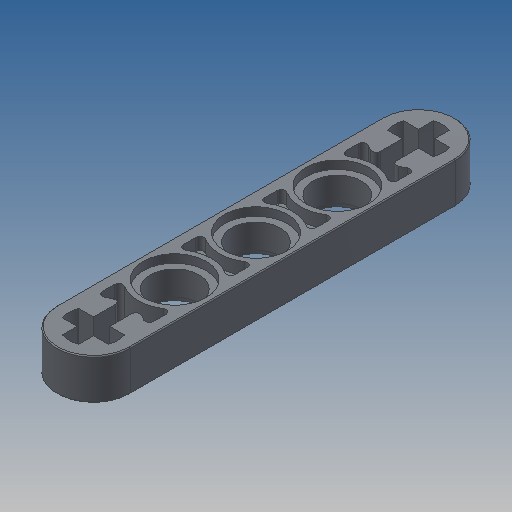
# Autodesk Inventor part: 11478-LtBluishGray
Saved by Autodesk Inventor 2022.2 (Build 262287010, 287A)
## iProperties
Created: 2012-03-21
Part Number: 11478-LtBluishGray
Document SubType Name: Modeling
Designer: D. Kohfeld
Density: 1.06 g/cm^3
Material: ABS Plastic
Mass: 0.640676 g
Surface Area: 12.0343 cm^2
Volume: 0.604411 cm^3
Appearance: LtBluishGray
Author: D. Kohfeld
Autodesk Inventor part; units mm, degrees
ref_plane "YZ Plane" through (0, 0, 0) normal (1, 0, 0) x (0, 1, 0)
ref_plane "XZ Plane" through (0, 0, 0) normal (0, 1, 0) x (-1, 0, 0)
ref_plane "XY Plane" through (0, 0, 0) normal (0, 0, 1) x (1, 0, 0)
sketch "Sketch1" plane through (0, 0, 0) normal (0, 0, 1) x (1, 0, 0)
  line L0 (3.6, -16) -> (3.6, 16)
  line L1 (-3.6, 16) -> (-3.6, -16)
  arc A0 (3.6, 16) -> (-3.6, 16) centre (0, 16) ccw
  circle A1 centre (0, 16) radius 2.4 construction
  circle A2 centre (0, 16) radius 3.2 construction
  circle A3 centre (0, 8) radius 3.2
  circle A4 centre (0, 8) radius 2.4
  line L2 (0, 8) -> (0, 16) construction
  line L3 (-2.5456, 13.4544) -> (-2.5456, 10.5456)
  line L4 (2.5456, 13.4544) -> (2.5456, 10.5456)
  arc A5 (-2.5456, 13.4544) -> (2.5456, 13.4544) centre (0, 16) ccw
  arc A6 (2.5456, 10.5456) -> (-2.5456, 10.5456) centre (0, 8) ccw
  arc A7 (-3.6, -16) -> (3.6, -16) centre (0, -16) ccw
  circle A8 centre (0, -16) radius 3.2 construction
  circle A9 centre (0, -16) radius 2.4 construction
  line L5 (-2.5456, -10.5456) -> (-2.5456, -13.4544)
  line L6 (2.5456, -10.5456) -> (2.5456, -13.4544)
  arc A10 (2.5456, -13.4544) -> (-2.5456, -13.4544) centre (0, -16) ccw
  line L7 (0.8, 12.49) -> (0.8, 15.2)
  line L8 (0.8, 15.2) -> (2.2627, 15.2)
  line L9 (2.2627, 16.8) -> (0.8, 16.8)
  line L10 (0.8, 16.8) -> (0.8, 18.2627)
  line L11 (-0.8, 18.2627) -> (-0.8, 16.8)
  line L12 (-0.8, 16.8) -> (-2.2627, 16.8)
  line L13 (-2.2627, 15.2) -> (-0.8, 15.2)
  line L14 (-0.8, 15.2) -> (-0.8, 12.49)
  arc A11 (-2.2627, 16.8) -> (-2.2627, 15.2) centre (0, 16) ccw
  arc A12 (0.8, 18.2627) -> (-0.8, 18.2627) centre (0, 16) ccw
  arc A13 (2.2627, 15.2) -> (2.2627, 16.8) centre (0, 16) ccw
  line L15 (-0.8, -18.2627) -> (-0.8, -16.8)
  line L16 (-0.8, -16.8) -> (-2.2627, -16.8)
  line L17 (-2.2627, -15.2) -> (-0.8, -15.2)
  line L18 (-0.8, -15.2) -> (-0.8, -12.49)
  line L19 (0.8, -12.49) -> (0.8, -15.2)
  line L20 (0.8, -15.2) -> (2.2627, -15.2)
  line L21 (2.2627, -16.8) -> (0.8, -16.8)
  line L22 (0.8, -16.8) -> (0.8, -18.2627)
  arc A14 (-2.2627, -15.2) -> (-2.2627, -16.8) centre (0, -16) ccw
  arc A15 (-0.8, -18.2627) -> (0.8, -18.2627) centre (0, -16) ccw
  arc A16 (2.2627, -16.8) -> (2.2627, -15.2) centre (0, -16) ccw
  circle A17 centre (0, 0) radius 3.2
  circle A18 centre (0, 0) radius 2.4
  circle A19 centre (0, -8) radius 3.2
  circle A20 centre (0, -8) radius 2.4
  line L23 (0, 8) -> (0, 0) construction
  line L24 (0, 0) -> (0, -8) construction
  line L25 (0, -8) -> (0, -16) construction
  line L26 (-2.5456, 13.4544) -> (0, 16) construction
  arc A21 (-2.5456, -10.5456) -> (2.5456, -10.5456) centre (0, -8) ccw
  line L27 (-2.5456, 5.4544) -> (-2.5456, 2.5456)
  line L28 (-2.5456, -2.5456) -> (-2.5456, -5.4544)
  line L29 (2.5456, -2.5456) -> (2.5456, -5.4544)
  line L30 (2.5456, 5.4544) -> (2.5456, 2.5456)
  arc A22 (-2.5456, 5.4544) -> (2.5456, 5.4544) centre (0, 8) ccw
  arc A23 (2.5456, 2.5456) -> (-2.5456, 2.5456) centre (0, 0) ccw
  arc A24 (-2.5456, -2.5456) -> (2.5456, -2.5456) centre (0, 0) ccw
  arc A25 (2.5456, -5.4544) -> (-2.5456, -5.4544) centre (0, -8) ccw
  dimension "d8" = 4.8
  dimension "d9" = 6.4
  dimension "d32" = 7.2
  dimension "d34" = 8
  dimension "d52" = 1.6
  dimension "d54" = 45
  constraints: 62 end point, 48 point on circle, 26 centre point, 23 equal radius, 18 equal length, 17 coincident, 14 parallel, 7 perpendicular, 7 vertical alignment, 5 collinear, 4 tangent, 3 vertical
  measures "d8" diameter of A1
  measures "d9" diameter of A2
  measures "d32" diameter of A0
  measures "d34" distance of L2.start L2.end
  measures "d52" distance between parallel lines of L10 L11
  measures "d54" angle of L1 L26
extrude "Extrusion1" add sketch "Sketch1" along normal mid plane 4 contours A7 L1 A0 L0 | A3 | A17 | A19
extrude "Extrusion9" add sketch "Sketch1" along normal mid plane 1.6 contours A22 L30 A23 L27 | A24 L29 A25 L28
sketch "Sketch6" plane through (0, 0, 2) normal (0, 0, 1) x (1, 0, 0)
  circle A0 centre (0, 8) radius 3.1
  circle A1 centre (0, 8) radius 2.4 projected
  arc A2 (2.5456, 2.5456) -> (-2.5456, 2.5456) centre (0, 0) ccw projected
  arc A3 (-2.5456, -10.5456) -> (2.5456, -10.5456) centre (0, -8) ccw projected
  circle A4 centre (0, 0) radius 3.1
  circle A5 centre (0, -8) radius 3.1
  dimension "d53" = 6.2
  constraints: 3 centre point, 2 coincident, 2 equal radius, 1 concentric
  measures "d53" diameter of A0
extrude "Extrusion7" cut sketch "Sketch6" against normal blind 0.8 contours A0 | A1 | A4 | A5
mirror "Mirror1" about plane through (0, 0, 0) normal (0, 0, 1) of "Extrusion7"
fillet "Fillet1" radius 0.1 6 edges at (0, 19.6, 2) (3.6, 0, 2) (-3.6, 0, 2) (0, 19.6, -2) (-3.6, 0, -2) (3.6, 0, -2)
fillet "Fillet1" radius 0.4 28 edges at (-2.5456, -10.5456, 0) (-2.5456, -13.4544, 0) (2.5456, -13.4544, 0) (2.5456, -10.5456, 0) (-2.5456, 13.4544, 0) (-2.5456, 10.5456, 0) (-0.8, -12.49, 0) (0.8, -12.49, 0) (2.5456, 10.5456, 0) (2.5456, 13.4544, 0) (0.8, 12.49, 0) (-0.8, 12.49, 0) (-2.5456, -5.4544, 1.4) (-2.5456, -2.5456, 1.4) (2.5456, -5.4544, 1.4) (2.5456, -2.5456, 1.4) (-2.5456, 2.5456, 1.4) (-2.5456, 5.4544, 1.4) (2.5456, 2.5456, 1.4) (2.5456, 5.4544, 1.4) (2.5456, -5.4544, -1.4) (2.5456, -2.5456, -1.4) (2.5456, 2.5456, -1.4) (2.5456, 5.4544, -1.4) (-2.5456, -5.4544, -1.4) (-2.5456, -2.5456, -1.4) (-2.5456, 2.5456, -1.4) (-2.5456, 5.4544, -1.4)
equation "\"d8\" = kd"
equation "\"d9\" = tsd"
equation "\"d32\" = tlad"
equation "\"d34\" = lu"
equation "\"d52\" = axlet"
equation "\"d14\" = 0.5 * lu"
equation "\"d55\" = wall"
equation "\"d41\" = tsl"
equation "\"kd\" = 4.8"
equation "\"tsd\" = 6.4"
equation "\"tlad\" = 7.2"
equation "\"lu\" = 8"
equation "\"axlet\" = 1.6"
equation "\"wall\" = 1.6"
equation "\"tsl\" = 0.8"
body "Solid1"
